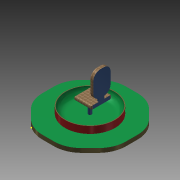
# Autodesk Inventor part: base
Saved by Autodesk Inventor 2015 (Build 190159000, 159)
## iProperties
Created: 2020-01-21
Part Number: base
Material: Aluminum 6061
Document SubType Name: Modeling
Designer: hp
Density: 2.7 g/cm^3
Appearance: Aluminum - Flat
Author: hp
Autodesk Inventor part; units mm, degrees
ref_plane "YZ Plane" through (0, 0, 0) normal (1, 0, 0) x (0, 1, 0)
ref_plane "XZ Plane" through (0, 0, 0) normal (0, 1, 0) x (-1, 0, 0)
ref_plane "XY Plane" through (0, 0, 0) normal (0, 0, 1) x (1, 0, 0)
sketch "Sketch1" plane through (0, 0, 0) normal (0, 1, 0) x (-1, 0, 0)
  line L0 (0, 19.6176) -> (898.0256, -878.408)
  line L1 (0, 19.6176) -> (1270, 19.6176) construction
  line L2 (0, 19.6176) -> (-1270, 19.6176)
  line L3 (-1270, 19.6176) -> (-2168.0256, -878.408)
  line L4 (-1270, 19.6176) -> (0, 19.6176) construction
  line L5 (898.0256, -878.408) -> (-2168.0256, -878.408)
  line L6 (898.0256, -878.408) -> (-2168.0256, -878.408)
  line L7 (-2168.0256, -878.408) -> (-2168.0256, -2148.408)
  line L8 (-2168.0256, -2148.408) -> (898.0256, -2148.408)
  line L9 (898.0256, -2148.408) -> (898.0256, -878.408)
  line L10 (898.0256, -2148.408) -> (0, -3046.4336)
  line L11 (898.0256, -2148.408) -> (2168.0256, -2148.408) construction
  line L12 (-2168.0256, -2148.408) -> (-1270, -3046.4336)
  line L13 (-1270, -3046.4336) -> (0, -3046.4336)
  point P0 (0, 0)
  dimension "d0" = 1270
  dimension "d1" = 45
  dimension "d2" = 1270
  dimension "d3" = 1270
  dimension "d4" = 135
  dimension "d5" = 1270
  dimension "d6" = 1270
  dimension "d7" = 135
  dimension "d8" = 1270
  constraints: 28 end point, 6 horizontal, 3 equal length, 2 parallel, 1 perpendicular
  measures "d0" distance of L0.start L0.end
  measures "d1" angle of L0 L1
  measures "d2" distance of L0.start L2.end
  measures "d3" distance of L2.end L3.end
  measures "d4" angle of L3 L4
  measures "d5" distance of L7.end L6.end
  measures "d6" distance of L8.end L10.end
  measures "d7" angle of L10 L11
  measures "d8" distance of L7.end L12.end
extrude "Extrusion1" add sketch "Sketch1" along normal blind 152.4
sketch "Sketch2" plane through (0, 152.4, 0) normal (0, 1, 0) x (1, 0, 0)
  circle A0 centre (623.2771, 1525.4657) radius 60.1528
  line L0 (2150.1664, 894.5684) -> (-903.6123, 2156.3631)
  line L1 (-903.6123, 2156.3631) -> (2150.1664, 2156.3631)
  line L2 (2150.1664, 2156.3631) -> (-903.6123, 894.5684)
  point P0 (0, 0)
  constraints: 6 end point, 2 midpoint, 1 centre point, 1 horizontal
extrude "Extrusion2" add sketch "Sketch2" along normal blind 508 contours A0 L0 L2 | L2 L0 A0 | A0 L2 L0 | L0 L2 A0
sketch "Sketch3" plane through (0, 152.4, 0) normal (0, 1, 0) x (1, 0, 0)
  point P0 (0, 0)
sketch "Sketch4" plane through (0, 152.4, 0) normal (0, 1, 0) x (1, 0, 0)
  line L0 (2168.5073, 886.5825) -> (-936.3093, 2164.3771)
  line L1 (-936.3093, 2164.3771) -> (2152.0565, 2164.3771)
  line L2 (2168.0256, 2148.408) -> (1270, 3046.4336) projected
  line L3 (2168.0256, 2148.408) -> (-889.8511, 886.5825)
  circle A0 centre (623.2771, 1525.4657) radius 60.1528 projected
  circle A1 centre (623.2771, 1525.4657) radius 914.8505
  circle A2 centre (623.2771, 1525.4657) radius 889.9971
  point P0 (0, 0)
  constraints: 6 end point, 2 centre point, 2 coincident, 1 horizontal, 1 point on line
extrude "Extrusion3" add sketch "Sketch4" along normal blind 254 contours A1 L3 A2 L0 | L0 A2 L3 A1 | A1 L0 A2 L3 | A1 L1 A2 L0 | L3 A2 L1 A1 | A1 L1 A2
sketch "Sketch5" plane through (623.2771, 660.4, -1525.4657) normal (0, 1, 0) x (1, 0, 0)
  line L0 (-623.2771, 370.6778) -> (424.0694, 370.6778)
  line L1 (424.0694, 370.6778) -> (424.0694, -382.2332)
  line L2 (424.0694, -382.2332) -> (-623.2771, -382.2332)
  line L3 (-623.2771, -382.2332) -> (-623.2771, 370.6778)
  line L4 (-623.2771, 370.6778) -> (-222.7925, 370.6778)
  line L5 (-222.7925, 370.6778) -> (-222.7925, -382.2332)
  line L6 (-222.7925, -382.2332) -> (-623.2771, -382.2332)
  line L7 (-623.2771, -382.2332) -> (-623.2771, 370.6778)
  point P0 (-623.2771, -1525.4657)
  constraints: 16 end point, 4 parallel, 2 horizontal, 2 perpendicular, 1 point on line
extrude "Extrusion4" add sketch "Sketch5" along normal blind 127 contours L0 L1 L2 L5
fillet "Fillet1" radius 50.8 10 edges at (723.9156, 787.4, -1143.2325) (723.9156, 787.4, -1896.1435) (1047.3465, 723.9, -1143.2325) (1047.3465, 723.9, -1896.1435) (400.4846, 787.4, -1519.688) (400.4846, 723.9, -1143.2325) (400.4846, 723.9, -1896.1435) (400.4846, 660.4, -1519.688) (723.9156, 660.4, -1143.2325) (723.9156, 660.4, -1896.1435)
sketch "Sketch6" plane through (623.2771, 787.4, -1525.4657) normal (0, 1, 0) x (1, 0, 0)
  line L0 (424.0694, -331.4332) -> (424.0694, 319.8778) projected
  line L1 (369.3973, -104.2761) -> (424.0694, -104.2761)
  line L2 (424.0694, -104.2761) -> (424.0694, 102.2791)
  line L3 (424.0694, 102.2791) -> (369.3973, 102.2791)
  line L4 (369.3973, 102.2791) -> (369.3973, -104.2761)
  point P0 (-623.2771, -1525.4657)
  constraints: 8 end point, 2 parallel, 1 horizontal, 1 perpendicular, 1 point on line
extrude "Extrusion5" add sketch "Sketch6" along normal blind 127
sketch "Sketch7" plane through (623.2771, 914.4, -1525.4657) normal (0, 1, 0) x (1, 0, 0)
  line L0 (424.0694, -331.4332) -> (-171.9925, -331.4332) projected
  line L1 (342.7048, -331.4332) -> (454.3712, -331.4332)
  line L2 (454.3712, -331.4332) -> (454.3712, 301.5078)
  line L3 (454.3712, 301.5078) -> (342.7048, 301.5078)
  line L4 (342.7048, 301.5078) -> (342.7048, -331.4332)
  point P0 (-623.2771, -1525.4657)
  constraints: 8 end point, 2 parallel, 1 horizontal, 1 perpendicular, 1 point on line
extrude "Extrusion6" add sketch "Sketch7" along normal blind 914.4
fillet "Fillet2" radius 254 4 edges at (1021.8151, 1828.8, -1194.0325) (1021.8151, 1828.8, -1826.9735) (1021.8151, 914.4, -1826.9735) (1021.8151, 914.4, -1194.0325)
fillet "Fillet3" radius 254 1 edges at (-266.72, 152.4, -1525.4657)
fillet "Fillet4" radius 1016 8 edges at (0, 76.2, 19.6176) (-898.0256, 76.2, -878.408) (-898.0256, 76.2, -2148.408) (0, 76.2, -3046.4336) (1270, 76.2, 19.6176) (2168.0256, 76.2, -878.408) (2168.0256, 76.2, -2148.408) (1270, 76.2, -3046.4336)
body "Solid1"
